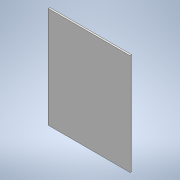
# Autodesk Inventor part: front_case
Saved by Autodesk Inventor 2022.1 (Build 261234020, 234B)
## iProperties
Created: 2022-02-06
Part Number: front_case
Material: Generic
Document SubType Name: Modeling
Designer: kee
Mass: 80.8099 g
Surface Area: 558.54 cm^2
Volume: 80.8099 cm^3
Density: 1 g/cm^3
Appearance: Default
Author: kee
Autodesk Inventor part; units mm, degrees
ref_plane "YZ Plane" through (0, 0, 0) normal (1, 0, 0) x (0, 1, 0)
ref_plane "XZ Plane" through (0, 0, 0) normal (0, 1, 0) x (-1, 0, 0)
ref_plane "XY Plane" through (0, 0, 0) normal (0, 0, 1) x (1, 0, 0)
sketch "Sketch1" plane through (0, 0, 0) normal (0, 0, 1) x (1, 0, 0)
  line L0 (-79.6424, 81.246) -> (67.8831, 81.246)
  line L1 (67.8831, 81.246) -> (67.8831, -101.3437)
  line L2 (67.8831, -101.3437) -> (-79.6424, -101.3437)
  line L3 (-79.6424, -101.3437) -> (-79.6424, 81.246)
  point P0 (0, 0)
  constraints: 8 end point, 2 parallel, 1 horizontal, 1 perpendicular
extrude "Extrusion1" add sketch "Sketch1" along normal blind 3
sketch "Sketch2" plane through (0, 0, 3) normal (0, 0, 1) x (1, 0, 0)
  point P0 (0, 0)
body "Solid1"
